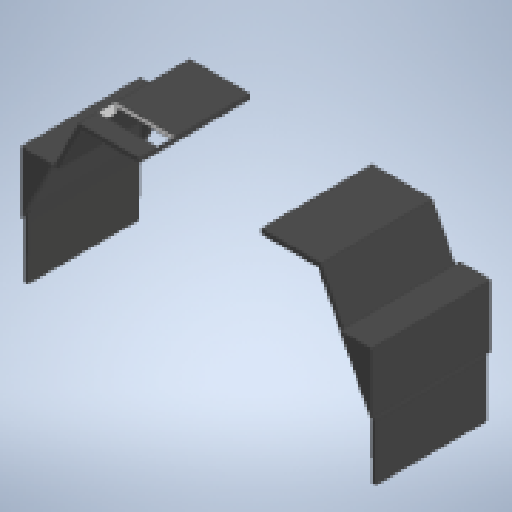
# Autodesk Inventor part: Middle sector
Saved by Autodesk Inventor 2024 (Build 280153000, 153)
## iProperties
Created: 2024-01-09
Part Number: Middle sector
Material: Generic
Document SubType Name: Modeling
Designer: Guru
Density: 1 g/cm^3
Appearance: Default
Author: Guru
Autodesk Inventor part; units mm, degrees
ref_plane "YZ Plane" through (0, 0, 0) normal (1, 0, 0) x (0, 1, 0)
ref_plane "XZ Plane" through (0, 0, 0) normal (0, 1, 0) x (-1, 0, 0)
ref_plane "XY Plane" through (0, 0, 0) normal (0, 0, 1) x (1, 0, 0)
ref_plane "Work Plane2" through (0, 0, 0) normal (0, 0, 1) x (1, 0, 0)
sketch "Sketch2" plane through (0, 0, 0) normal (0, 0, 1) x (1, 0, 0)
  line L0 (162.4366, 63.866) -> (234.4261, -79.7039) projected
  line L1 (241.4222, -79.4895) -> (177.7412, 47.5105) projected
  line L2 (-228.4778, -3.2895) -> (228.7222, -3.2895) projected
  line L3 (228.7222, -3.2895) -> (228.7222, -54.0895) projected
  line L4 (-228.4778, -3.2895) -> (-228.4778, -54.0895) projected
  line L5 (241.4222, -155.6895) -> (241.4222, -79.4895) projected
  line L6 (241.4222, -79.4895) -> (166.3561, 70.216) projected
  line L7 (166.3561, 70.216) -> (77.4561, 70.216) projected
  line L8 (77.4561, 70.216) -> (77.4561, 47.5105) projected
  line L9 (77.4561, 47.5105) -> (-77.2118, 47.5105) projected
  line L10 (-77.2118, 47.5105) -> (-77.2118, 70.216) projected
  line L11 (-77.2118, 70.216) -> (-166.1118, 70.216) projected
  line L12 (-166.1118, 70.216) -> (-241.1778, -79.4895) projected
  line L13 (-241.1778, -79.4895) -> (-241.1778, -155.6895) projected
  line L14 (-241.1778, -155.6895) -> (-233.8379, -155.6895) projected
  line L15 (-233.8379, -155.6895) -> (-231.9549, -75.263) projected
  line L16 (-231.9549, -75.263) -> (-162.1922, 63.866) projected
  line L17 (-162.1922, 63.866) -> (-83.5618, 63.866) projected
  line L18 (-83.5618, 63.866) -> (-83.5618, 41.1605) projected
  line L19 (-83.5618, 41.1605) -> (83.8061, 41.1605) projected
  line L20 (83.8061, 41.1605) -> (83.8061, 63.866) projected
  line L21 (83.8061, 63.866) -> (162.4366, 63.866) projected
  line L22 (162.4366, 63.866) -> (234.4261, -79.7039) projected
  line L23 (234.4261, -79.7039) -> (236.2052, -155.6895) projected
  line L24 (236.2052, -155.6895) -> (241.4222, -155.6895) projected
  line L25 (233.8022, -54.0895) -> (233.8022, 1.7905)
  line L26 (233.8022, 1.7905) -> (-233.5578, 1.7905)
  line L27 (-233.5578, 1.7905) -> (-233.5578, -54.0895)
  line L28 (240.1522, -54.0895) -> (240.1522, 8.1405)
  line L29 (240.1522, 8.1405) -> (-239.9078, 8.1405)
  line L30 (-239.9078, 8.1405) -> (-239.9078, -54.0895)
  line L31 (233.8022, -54.0895) -> (233.8022, -64.2928)
  line L32 (240.1522, -54.0895) -> (240.1522, -76.9567)
  line L33 (233.8022, -64.2928) -> (234.0782, -64.8433)
  line L34 (240.1522, -76.9567) -> (241.4222, -79.4895)
  line L35 (241.4222, -79.4895) -> (241.4222, -155.6895)
  line L36 (241.4222, -155.6895) -> (236.2052, -155.6895)
  line L37 (236.2052, -155.6895) -> (234.4261, -79.7039)
  line L38 (233.8022, -64.2928) -> (234.4261, -79.7039)
  line L39 (83.8061, 63.866) -> (83.8061, 70.216)
  point P0 (0, 0)
  point P1 (197.4823, 8.1405)
  point P2 (193.5628, 1.7905)
  dimension "d0" = 5.08
  dimension "d1" = 6.35
  constraints: 30 end point, 5 point on line, 4 collinear, 2 perpendicular, 1 parallel, 4 other
  measures "d0" distance between parallel lines of L2 L26
  measures "d1" distance between parallel lines of L25 L28
ref_plane "Work Plane3" through (-241.1778, -155.6895, 152.4) normal (0, 0, -1) x (0, 1, 0)
extrude "Extrusion1" add sketch "Sketch2" along normal up to surface (152.4 mm away) contours L21 L39 L7 L6 L1 L29 L0 | L29 L1 L26 L0 | L29 L28 L32 L1 L31 L25 L26 | L38 L1 L5 L24 L23
sketch "Sketch3" plane through (83.8061, 70.216, 152.4) normal (0, 0, 1) x (1, 0, 0)
  line L0 (156.3461, -62.0755) -> (113.6762, -62.0755) projected
  line L1 (156.3461, -147.1727) -> (156.3461, -62.0755) projected
  line L2 (113.6762, -62.0755) -> (156.3461, -62.0755)
  line L3 (157.6161, -149.7055) -> (156.3461, -147.1727) projected
  line L4 (156.3461, -62.0755) -> (156.3461, -147.1727)
  line L5 (156.3461, -147.1727) -> (116.8602, -68.4255)
  line L6 (109.7567, -68.4255) -> (149.9961, -68.4255) projected
  line L7 (113.6762, -62.0755) -> (116.8602, -68.4255)
  point P0 (-83.8061, -70.216)
  constraints: 8 end point, 2 perpendicular, 1 collinear, 1 point on line
extrude "Extrusion2" add sketch "Sketch3" along normal blind 5.08
sketch "Sketch4" plane through (0, 0, 0) normal (0, 0, -1) x (-1, 0, 0)
  line L0 (-240.1522, 8.1405) -> (-197.4823, 8.1405) projected
  line L1 (-240.1522, -76.9567) -> (-240.1522, 8.1405) projected
  line L2 (-233.8022, 1.7905) -> (-233.8022, -64.2928) projected
  line L3 (-241.4222, -79.4895) -> (-177.7412, 47.5105) projected
  line L4 (-193.5628, 1.7905) -> (-233.8022, 1.7905) projected
  line L5 (-241.4222, -79.4895) -> (-177.7412, 47.5105) projected
  line L6 (-240.1522, -76.9567) -> (-197.4823, 8.1405)
  line L7 (-240.1522, 8.1405) -> (-197.4823, 8.1405)
  line L8 (-240.1522, 8.1405) -> (-240.1522, -76.9567)
  point P0 (0, 0)
  constraints: 6 end point, 1 collinear, 1 perpendicular
extrude "Extrusion3" add sketch "Sketch4" along normal blind 6.35
chamfer "Chamfer2" distance 2.54 angle 45 1 edges at (240.1522, -76.9567, 76.2)
mirror "Mirror1" about plane through (0, 0, 0) normal (1, 0, 0) of "Extrusion1", "Extrusion3", "Extrusion2"
sketch "Sketch5" plane through (-166.3561, 70.216, 0) normal (0, 1, 0) x (1, 0, 0)
  line L0 (82.55, 0) -> (82.55, -152.4) projected
  line L1 (82.55, -98.2218) -> (173.9777, -98.2218)
  line L2 (173.9777, -98.2218) -> (173.9777, -130.3782)
  line L3 (173.9777, -130.3782) -> (82.55, -130.3782)
  line L4 (82.55, -130.3782) -> (82.55, -98.2218)
  line L5 (73.0499, -104.5718) -> (98.4499, -104.5718) projected
  line L6 (73.0499, -124.0282) -> (98.4499, -124.0282) projected
  point P0 (166.3561, 0)
  dimension "d14" = 6.35
  dimension "d15" = 6.35
  constraints: 8 end point, 2 parallel, 1 horizontal, 1 perpendicular, 1 point on line
  measures "d14" distance between parallel lines of L5 L1
  measures "d15" distance between parallel lines of L3 L6
extrude "Extrusion5" cut sketch "Sketch5" against normal blind 50.8
sketch "Sketch6" plane through (-166.3561, 70.216, 0) normal (0, 1, 0) x (1, 0, 0)
  line L0 (-62.1217, -101.6) -> (395.0783, -101.6) projected
  line L1 (90.2783, -124.0282) -> (109.3283, -124.0282) projected
  line L2 (90.2783, -129.1082) -> (90.2783, -124.0282) projected
  line L3 (109.3283, -129.1082) -> (90.2783, -129.1082) projected
  line L4 (109.3283, -124.0282) -> (109.3283, -129.1082) projected
  line L5 (-62.1217, -127) -> (395.0783, -127) projected
  line L6 (0, 0) -> (0, -152.4) projected
  line L7 (82.4528, -101.6) -> (0, -101.6)
  line L8 (0, -101.6) -> (0, -127)
  line L9 (0, -127) -> (82.4528, -127)
  line L10 (82.4528, -127) -> (82.4528, -101.6)
  point P0 (166.3561, 0)
  point P1 (0, -101.6)
  constraints: 8 end point, 3 point on line, 2 parallel, 1 horizontal, 1 perpendicular
extrude "Extrusion6" cut sketch "Sketch6" against normal blind 50.8 contours L0 L10 L5 L6
sketch "Sketch7" plane through (-83.8061, 63.866, 0) normal (1, 0, 0) x (0, 0, -1)
  line L0 (-127, 0) -> (-101.6, 0) projected
  line L1 (-127, 6.35) -> (-127, 0) projected
  line L2 (-101.6, 6.35) -> (-127, 6.35) projected
  line L3 (-101.6, 6.35) -> (-101.6, 0) projected
  line L4 (-127, 6.35) -> (-101.6, 6.35)
  line L5 (-101.6, 6.35) -> (-101.6, 0)
  line L6 (-101.6, 0) -> (-127, 0)
  line L7 (-127, 0) -> (-127, 6.35)
  point P0 (0, -63.866)
  constraints: 8 end point, 2 parallel, 1 horizontal, 1 perpendicular
extrude "Extrusion7" cut sketch "Sketch7" against normal blind 50.8
body "Solid1"
